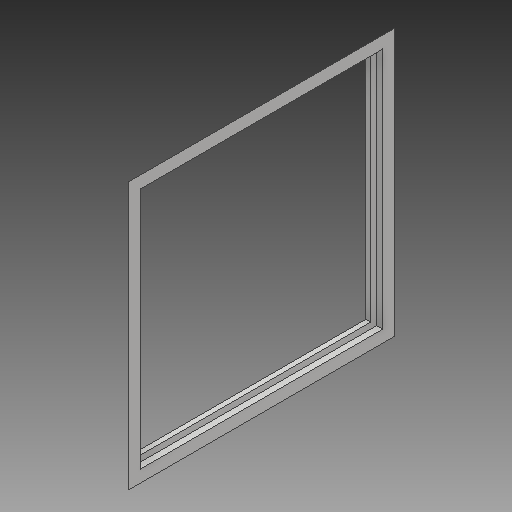
# Autodesk Inventor part: PV_Rahmen_CPY2
Saved by Autodesk Inventor 2018.3 (Build 223284000, 284)
## iProperties
Created: 2019-11-04
Part Number: PV_Rahmen_CPY2
Material: Generisch
Document SubType Name: Modeling
Designer: DerLobre
Density: 1 g/cm^3
Appearance: Vorgabe
Author: DerLobre
Autodesk Inventor part; units mm, degrees
ref_plane "YZ Plane" through (0, 0, 0) normal (1, 0, 0) x (0, 1, 0)
ref_plane "XZ Plane" through (0, 0, 0) normal (0, 1, 0) x (-1, 0, 0)
ref_plane "XY Plane" through (0, 0, 0) normal (0, 0, 1) x (1, 0, 0)
sketch "Skizze1" plane through (0, 0, 0) normal (1, 0, 0) x (0, 1, 0)
  line L0 (-230.3873, 208.9718) -> (209.6127, 208.9718)
  line L1 (209.6127, 208.9718) -> (209.6127, -231.0282)
  line L2 (209.6127, -231.0282) -> (-230.3873, -231.0282)
  line L3 (-230.3873, -231.0282) -> (-230.3873, 208.9718)
  point P0 (0, 0)
  dimension "d0" = 440
  dimension "d1" = 440
  constraints: 8 end point, 2 parallel, 1 horizontal, 1 perpendicular
  measures "d0" distance of L0.start L0.end
  measures "d1" distance of L2.end L0.start
extrude "Extrusion1" add sketch "Skizze1" along normal blind 18
sketch "Skizze2" plane through (18, 0, 0) normal (1, 0, 0) x (0, 0, -1)
  line L0 (-208.9718, 209.6127) -> (-208.9718, -230.3873) projected
  line L1 (-208.9718, -230.3873) -> (231.0282, -230.3873) projected
  line L2 (231.0282, -230.3873) -> (231.0282, 209.6127) projected
  line L3 (231.0282, 209.6127) -> (-208.9718, 209.6127) projected
  line L4 (-188.9718, -210.3873) -> (211.0282, -210.3873)
  line L5 (211.0282, -210.3873) -> (211.0282, 189.6127)
  line L6 (211.0282, 189.6127) -> (-188.9718, 189.6127)
  line L7 (-188.9718, 189.6127) -> (-188.9718, -210.3873)
  point P0 (0, 0)
  dimension "d4" = 20
  dimension "d5" = 20
  dimension "d6" = 20
  dimension "d7" = 20
  constraints: 8 end point, 2 parallel, 1 horizontal, 1 perpendicular
  measures "d4" distance between parallel lines of L2 L5
  measures "d5" distance between parallel lines of L3 L6
  measures "d6" distance between parallel lines of L0 L7
  measures "d7" distance between parallel lines of L1 L4
extrude "Extrusion2" cut sketch "Skizze2" against normal blind 10 contours L7 L6 L5 L4
sketch "Skizze3" plane through (8, 0, 0) normal (1, 0, 0) x (0, 0, -1)
  line L0 (211.0282, -210.3873) -> (-188.9718, -210.3873) projected
  line L1 (211.0282, 189.6127) -> (211.0282, -210.3873) projected
  line L2 (-188.9718, 189.6127) -> (211.0282, 189.6127) projected
  line L3 (-188.9718, -210.3873) -> (-188.9718, 189.6127) projected
  line L4 (-178.9718, -200.3873) -> (201.0282, -200.3873)
  line L5 (201.0282, -200.3873) -> (201.0282, 179.6127)
  line L6 (201.0282, 179.6127) -> (-178.9718, 179.6127)
  line L7 (-178.9718, 179.6127) -> (-178.9718, -200.3873)
  point P0 (0, 0)
  dimension "d10" = 10
  dimension "d11" = 10
  dimension "d12" = 10
  dimension "d13" = 10
  constraints: 8 end point, 2 parallel, 1 horizontal, 1 perpendicular
  measures "d10" distance between parallel lines of L1 L5
  measures "d11" distance between parallel lines of L2 L6
  measures "d12" distance between parallel lines of L3 L7
  measures "d13" distance between parallel lines of L0 L4
extrude "Extrusion3" cut sketch "Skizze3" against normal blind 8 contours L7 L6 L5 L4
sketch "Skizze6" plane through (0, 0, 0) normal (-1, 0, 0) x (0, 0, 1)
  line L0 (-201.0282, -200.3873) -> (-201.0282, 179.6127) projected
  line L1 (-201.0282, 179.6127) -> (178.9718, 179.6127) projected
  line L2 (178.9718, 179.6127) -> (178.9718, -200.3873) projected
  line L3 (178.9718, -200.3873) -> (-201.0282, -200.3873) projected
  line L4 (208.9718, -230.3873) -> (208.9718, 209.6127) projected
  line L5 (208.9718, 209.6127) -> (-231.0282, 209.6127) projected
  line L6 (-231.0282, 209.6127) -> (-231.0282, -230.3873) projected
  line L7 (-231.0282, -230.3873) -> (208.9718, -230.3873) projected
  line L8 (6.4718, -214.3873) -> (6.4718, -223.3873) projected
  line L9 (10.9718, -214.3873) -> (6.4718, -214.3873) projected
  line L10 (6.4718, -223.3873) -> (1.9718, -223.3873) projected
  line L11 (1.9718, -210.3873) -> (1.9718, -223.3873) projected
  line L12 (10.9718, -210.3873) -> (10.9718, -214.3873) projected
  line L13 (-211.0282, -210.3873) -> (188.9718, -210.3873) projected
  line L14 (-0.0282, -210.3873) -> (-0.0282, -223.3873) projected
  line L15 (-9.0282, -210.3873) -> (-9.0282, -214.3873) projected
  line L16 (-4.5282, -214.3873) -> (-9.0282, -214.3873) projected
  line L17 (-4.5282, -214.3873) -> (-4.5282, -223.3873) projected
  line L18 (-0.0282, -223.3873) -> (-4.5282, -223.3873) projected
  line L19 (-16.0282, -210.3873) -> (-16.0282, -214.3873) projected
  line L20 (-16.0282, -214.3873) -> (-20.5282, -214.3873) projected
  line L21 (-20.5282, -214.3873) -> (-20.5282, -223.3873) projected
  line L22 (-20.5282, -223.3873) -> (-25.0282, -223.3873) projected
  line L23 (-25.0282, -210.3873) -> (-25.0282, -223.3873) projected
  line L24 (-27.0282, -210.3873) -> (-27.0282, -223.3873) projected
  line L25 (-27.0282, -223.3873) -> (-31.5282, -223.3873) projected
  line L26 (-31.5282, -214.3873) -> (-31.5282, -223.3873) projected
  line L27 (-31.5282, -214.3873) -> (-36.0282, -214.3873) projected
  line L28 (-36.0282, -210.3873) -> (-36.0282, -214.3873) projected
  line L29 (-231.0282, -230.3873) -> (208.9718, -230.3873) projected
  line L30 (14.0665, -230.3873) -> (14.0665, -200.3873)
  line L31 (-39.201, -230.3873) -> (-39.201, -200.3873)
  point P0 (0, 0)
  constraints: 4 end point, 4 point on line, 2 perpendicular, 1 other
extrude "Extrusion4" cut sketch "Skizze6" against normal blind 15 contours L3 L30 L13 L31 | L13 L28 L27 L26 L25 L24 L23 L22 L21 L20 L19 L15 L16 L17 L18 L14 L11 L10 L8 L9 L12 L30 L7 L31 | L13 L24 L25 L26 L27 L28 | L12 L9 L8 L10 L11 L13 | L13 L19 L20 L21 L22 L23 | L14 L18 L17 L16 L15 L13
chamfer "Fase1" distance 18 angle 45 1 edges at (0, -230.3873, 111.5191)
chamfer "Fase2" distance 18 angle 45 2 edges at (0, 209.6127, -11.0282) (0, -1.3876, 208.9718)
